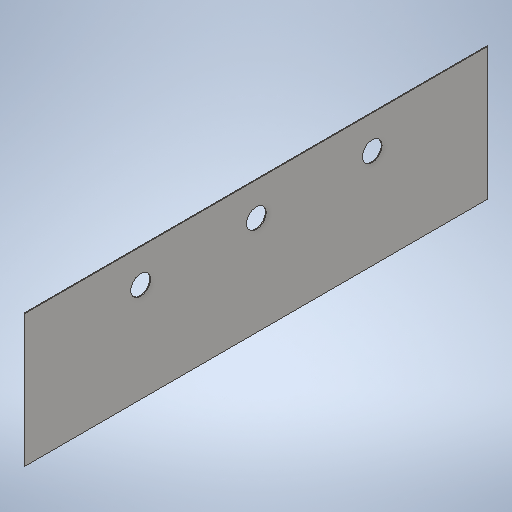
# Autodesk Inventor part: project support plate small
Saved by Autodesk Inventor 2025.2 (Build 292293000, 293)
## iProperties
Created: 2025-02-04
Part Number: project support plate small
Material: Steel, Galvanized
Document SubType Name: Sheet Metal
Designer: nandu
Density: 7.85 g/cm^3
Sheet Metal Rule: Default
Appearance: Galvanized
Author: nandu
Autodesk Inventor part; units mm, degrees
ref_plane "YZ Plane" through (0, 0, 0) normal (1, 0, 0) x (0, 1, 0)
ref_plane "XZ Plane" through (0, 0, 0) normal (0, 1, 0) x (-1, 0, 0)
ref_plane "XY Plane" through (0, 0, 0) normal (0, 0, 1) x (1, 0, 0)
sketch "Sketch1" plane through (0, 0, 0) normal (1, 0, 0) x (0, 1, 0)
  line L0 (0, 0) -> (100, 0)
  line L1 (100, 0) -> (100, -350)
  line L2 (100, -350) -> (0, -350)
  line L3 (0, -350) -> (0, 0)
  dimension "d0" = 100
  dimension "d1" = 350
  constraints: 8 end point, 2 parallel, 1 horizontal, 1 perpendicular
  measures "d0" distance of L1.end L2.end
  measures "d1" distance of L0.end L1.end
extrude "Extrusion1" add sketch "Sketch1" along normal blind 0.607
sketch "Sketch2" plane through (0.607, 0, 0) normal (1, 0, 0) x (0, 0, -1)
  line L0 (350, 100) -> (0, 100) projected
  line L1 (0, 100) -> (175, 100)
  line L2 (175, 100) -> (175, 75)
  circle A0 centre (175, 75) radius 7.5
  line L3 (175, 75) -> (87.5, 75)
  line L4 (175, 75) -> (262.5, 75)
  circle A1 centre (87.5, 75) radius 7.5
  circle A2 centre (262.5, 75) radius 7.5
  point P0 (0, 0)
  dimension "d4" = 175
  dimension "d5" = 25
  dimension "d6" = 15
  dimension "d10" = 15
  dimension "d11" = 15
  dimension "d12" = 87.5
  constraints: 8 end point, 3 centre point, 3 coincident, 2 horizontal, 1 midpoint, 1 vertical
  measures "d4" distance of L0.end L1.end
  measures "d5" distance of L1.end L2.end
  measures "d6" diameter of A0
  measures "d10" diameter of A1
  measures "d11" diameter of A2
  measures "d12" distance of L3.end L2.end
extrude "Extrusion2" cut sketch "Sketch2" against normal through all
equation "\"BendRadius\" = Thickness"
equation "\"BendReliefWidth\" = Thickness"
equation "\"BendReliefDepth\" = 0.5 * Thickness"
equation "\"CornerReliefSize\" = 4 * Thickness"
equation "\"MinimumRemnant\" = 2 * Thickness"
equation "\"TransitionRadius\" = BendRadius"
equation "\"JacobiRadiusSize\" = BendRadius"
equation "\"GapSize\" = Thickness"
equation "\"Thickness\" = 3.048"
body "Solid1"
